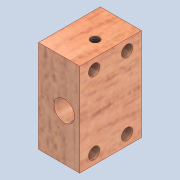
# Autodesk Inventor part: 0005-10-015 suport tija
Saved by Autodesk Inventor 2020 (Build 240168000, 168)
## iProperties
Created: 2020-12-19
Part Number: 0005-10-015 suport tija
Material: Wood (Maple)
Document SubType Name: Modeling
Designer: Iulian Bors
Density: 0.67 g/cm^3
Appearance: Red Oak - Natural Low Gloss
Mass: 14.9073 g
Surface Area: 80.9945 cm^2
Volume: 22.2498 cm^3
Author: Iulian Bors
Subject: 015
Autodesk Inventor part; units mm, degrees
ref_plane "YZ Plane" through (0, 0, 0) normal (1, 0, 0) x (0, 1, 0)
ref_plane "XZ Plane" through (0, 0, 0) normal (0, 1, 0) x (-1, 0, 0)
ref_plane "XY Plane" through (0, 0, 0) normal (0, 0, 1) x (1, 0, 0)
sketch "Sketch1" plane through (0, 0, 0) normal (0, 0, 1) x (1, 0, 0)
  line L0 (-10, 22.5) -> (10, 22.5)
  line L1 (10, 22.5) -> (10, -22.5)
  line L2 (10, -22.5) -> (-10, -22.5)
  line L3 (-10, -22.5) -> (-10, 22.5)
  point P0 (0, 0)
  point P1 (0, 22.5)
  point P2 (-10, 0)
  dimension "d0" = 20
  dimension "d1" = 45
  constraints: 8 end point, 2 midpoint, 2 parallel, 1 horizontal, 1 horizontal alignment, 1 perpendicular, 1 vertical alignment
  measures "d0" distance of L0.start L0.end
  measures "d1" distance of L0.end L1.end
extrude "Extrusion1" add sketch "Sketch1" along normal blind 30
sketch "Sketch3" plane through (0, 0, 0) normal (0, 0, -1) x (-1, 0, 0)
  circle A0 centre (-2.5, 0) radius 5
  line L0 (-10, -22.5) -> (-10, 22.5) projected
  point P0 (-10, 0)
  dimension "d4" = 10
  dimension "d5" = 7.5
  constraints: 1 centre point, 1 horizontal alignment, 1 midpoint
  measures "d4" diameter of A0
  measures "d5" distance from line of A0.centre L0
extrude "Extrusion2" cut sketch "Sketch3" against normal through all
sketch "Sketch4" plane through (10, -22.5, 0) normal (1, 0, 0) x (0, 0, -1)
  circle A0 centre (-7, 40) radius 2.75
  circle A1 centre (-7, 5) radius 2.75
  line L0 (0, 0) -> (0, 45) projected
  line L1 (0, 45) -> (-30, 45) projected
  line L2 (0, 0) -> (-30, 0) projected
  circle A2 centre (-23, 40) radius 2.75
  circle A3 centre (-23, 5) radius 2.75
  line L3 (-30, 0) -> (-30, 45) projected
  point P0 (0, 22.5)
  dimension "d8" = 5.5
  dimension "d9" = 5.5
  dimension "d10" = 7
  dimension "d11" = 5
  dimension "d12" = 5
  dimension "d13" = 7
  dimension "d16" = 35
  dimension "d17" = 16
  constraints: 4 centre point, 2 equal radius, 2 horizontal alignment, 2 vertical alignment
  measures "d8" diameter of A0
  measures "d9" diameter of A1
  measures "d10" distance from line of L0 A0.centre
  measures "d11" distance from line of A0.centre L1
  measures "d12" distance from line of L2 A1.centre
  measures "d13" distance from line of L3 A2.centre
  measures "d16" distance of A0.centre A1.centre
  measures "d17" distance of A3.centre A1.centre
extrude "Extrusion3" cut sketch "Sketch4" against normal through all contours A1
pattern_linear "Rectangular Pattern1" count 2 spacing 16 along (0, 0, 1) count 2 spacing 35 along (0, 1, 0) of "Extrusion3"
sketch "Sketch5" plane through (-10, -22.5, 0) normal (0, -1, 0) x (1, 0, 0)
  line L0 (0, 0) -> (0, 30) projected
  line L1 (0, 0) -> (20, 0) projected
  point P0 (12.5, 15)
  point P1 (0, 15)
  point P2 (10, 0)
  dimension "d38" = 12.5
  constraints: 2 midpoint, 1 horizontal alignment
  measures "d38" distance from line of L0 point (12.5, 15)
hole "Hole1" at (2.5, -22.5, 15) direction (0, 1, 0) diameter 4.134 end through all thread size "M5x0.8" class "6H" standard "ISO Metric profile"
equation "\"d13\" = d10"
body "Solid1"
